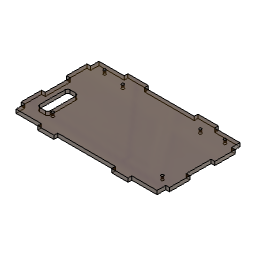
PCB Plate (Autodesk Fusion 360 design; units mm, degrees)
Autodesk Fusion 360 part; units mm, degrees
sketch "Sketch1" plane through (0, 0, 0) normal (0, 0, 1) x (1, 0, 0)
  line L0 (90, -52.5) -> (-90, -52.5)
  line L1 (-90, -52.5) -> (-90, 52.5)
  line L2 (-90, 52.5) -> (90, 52.5)
  line L3 (90, 52.5) -> (90, -52.5)
  line L4 (90, -52.5) -> (-90, 52.5) construction
  line L5 (-90, -52.5) -> (90, 52.5) construction
  line L6 (-85.5, 52.5) -> (-85.5, -52.5)
  line L7 (85.5, 52.5) -> (85.5, -52.5)
  line L8 (-90, -48) -> (90, -48)
  line L9 (-90, -52.5) -> (-55, -52.5)
  line L10 (-55, -52.5) -> (-55, -48)
  line L11 (-55, -48) -> (-90, -48)
  line L12 (-90, -48) -> (-90, -52.5)
  line L13 (-55, -52.5) -> (-35, -52.5)
  line L14 (-35, -52.5) -> (-35, -48)
  line L15 (-35, -48) -> (-55, -48)
  line L16 (-55, -48) -> (-55, -52.5)
  line L17 (90, -52.5) -> (55, -52.5)
  line L18 (55, -52.5) -> (55, -48)
  line L19 (55, -48) -> (90, -48)
  line L20 (90, -48) -> (90, -52.5)
  line L21 (-90, -52.5) -> (-85.5, -52.5)
  line L22 (-85.5, -52.5) -> (-85.5, -37.5)
  line L23 (-85.5, -37.5) -> (-90, -37.5)
  line L24 (-90, -37.5) -> (-90, -52.5)
  line L25 (90, -52.5) -> (85.5, -52.5)
  line L26 (85.5, -52.5) -> (85.5, -37.5)
  line L27 (85.5, -37.5) -> (90, -37.5)
  line L28 (90, -37.5) -> (90, -52.5)
  line L29 (-85.5, -37.5) -> (-90, -37.5)
  line L30 (-90, -37.5) -> (-90, -12.5)
  line L31 (-90, -12.5) -> (-85.5, -12.5)
  line L32 (-85.5, -12.5) -> (-85.5, -37.5)
  line L33 (90, -37.5) -> (85.5, -37.5)
  line L34 (85.5, -37.5) -> (85.5, -12.5)
  line L35 (85.5, -12.5) -> (90, -12.5)
  line L36 (90, -12.5) -> (90, -37.5)
  line L37 (-85.5, -12.5) -> (-90, -12.5)
  line L38 (-90, -12.5) -> (-90, 17.5)
  line L39 (-90, 17.5) -> (-85.5, 17.5)
  line L40 (-85.5, 17.5) -> (-85.5, -12.5)
  line L41 (-85.5, 17.5) -> (-90, 17.5)
  line L42 (-90, 17.5) -> (-90, 42.5)
  line L43 (-90, 42.5) -> (-85.5, 42.5)
  line L44 (-85.5, 42.5) -> (-85.5, 17.5)
  line L45 (90, -12.5) -> (85.5, -12.5)
  line L46 (85.5, -12.5) -> (85.5, 17.5)
  line L47 (85.5, 17.5) -> (90, 17.5)
  line L48 (90, 17.5) -> (90, -12.5)
  line L49 (90, 17.5) -> (85.5, 17.5)
  line L50 (85.5, 17.5) -> (85.5, 42.5)
  line L51 (85.5, 42.5) -> (90, 42.5)
  line L52 (90, 42.5) -> (90, 17.5)
  line L53 (55, -52.5) -> (35, -52.5)
  line L54 (35, -52.5) -> (35, -48)
  line L55 (35, -48) -> (55, -48)
  line L56 (55, -48) -> (55, -52.5)
  line L57 (-90, 43) -> (90, 43) construction
  line L58 (0, 43) -> (0, 40) construction
  circle A0 centre (47, 43) radius 1.6
  circle A1 centre (-47, 43) radius 1.6
  line L59 (-90, 47) -> (90, 47) construction
  circle A2 centre (73, 47) radius 1.6
  circle A3 centre (-73, 47) radius 1.6
  circle A4 centre (73, -29) radius 1.6
  circle A5 centre (-60, -29) radius 1.6
  line L60 (-66, -32) -> (-73, -32)
  line L61 (-76, -29) -> (-76, 2)
  line L62 (-73, 5) -> (-66, 5)
  line L63 (-63, 2) -> (-63, -29)
  line L64 (-63, -32) -> (-76, 5) construction
  line L65 (-76, -32) -> (-63, 5) construction
  arc A6 (-63, 2) -> (-66, 5) centre (-66, 2) ccw
  arc A7 (-73, 5) -> (-76, 2) centre (-73, 2) ccw
  arc A8 (-76, -29) -> (-73, -32) centre (-73, -29) ccw
  arc A9 (-66, -32) -> (-63, -29) centre (-66, -29) ccw
  line L66 (-55, 52.5) -> (-30, 52.5)
  line L67 (-30, 52.5) -> (-30, 57)
  line L68 (-30, 57) -> (-55, 57)
  line L69 (-55, 57) -> (-55, 52.5)
  line L70 (30, 52.5) -> (55, 52.5)
  line L71 (55, 52.5) -> (55, 57)
  line L72 (55, 57) -> (30, 57)
  line L73 (30, 57) -> (30, 52.5)
  point P0 (-69.5, -13.5)
  dimension "d1" = 180
  dimension "d2" = 105
  dimension "d3" = 4.5
  dimension "d4" = 4.5
  dimension "d5" = 4.5
  dimension "d6" = 35
  dimension "d7" = 20
  dimension "d8" = 35
  dimension "d10" = 15
  dimension "d11" = 15
  dimension "d12" = 25
  dimension "d13" = 25
  dimension "d14" = 30
  dimension "d15" = 25
  dimension "d16" = 30
  dimension "d17" = 25
  dimension "d18" = 20
  dimension "d20" = 91
  dimension "d21" = 3.2
  dimension "d22" = 3.2
  dimension "d23" = 47
  dimension "d24" = 47
  dimension "d25" = 4
  dimension "d26" = 3.2
  dimension "d27" = 3.2
  dimension "d28" = 73
  dimension "d29" = 73
  dimension "d30" = 3.2
  dimension "d31" = 72
  dimension "d32" = 3.2
  dimension "d33" = 72
  dimension "d34" = 60
  dimension "d35" = 13
  dimension "d36" = 37
  dimension "d37" = 3
  dimension "d38" = 3
  dimension "d39" = 3
  dimension "d40" = 3
  dimension "d41" = 3
  dimension "d42" = 3
  dimension "d48" = 25
  dimension "d49" = 4.5
  dimension "d50" = 25
  dimension "d51" = 4.5
  dimension "d52" = 35
  dimension "d53" = 35
  constraint horizontal L0
  constraint perpendicular L0 L1
  constraint parallel L0 L2
  constraint parallel L1 L3
  constraint coincident L4 origin
  constraint coincident L5 origin
  constraint coincident L2 L6.start
  constraint coincident L0 L6.end
  constraint perpendicular L0 L6
  constraint coincident L2 L7.start
  constraint coincident L0 L7.end
  constraint perpendicular L0 L7
  constraint coincident L1 L8.start
  constraint coincident L3 L8.end
  constraint perpendicular L3 L8
  constraint horizontal L9
  constraint vertical L10
  constraint horizontal L11
  constraint vertical L12
  constraint horizontal L13
  constraint vertical L14
  constraint horizontal L15
  constraint vertical L16
  constraint horizontal L17
  constraint vertical L18
  constraint horizontal L19
  constraint vertical L20
  constraint horizontal L21
  constraint vertical L22
  constraint horizontal L23
  constraint vertical L24
  constraint horizontal L25
  constraint vertical L26
  constraint horizontal L27
  constraint vertical L28
  constraint horizontal L29
  constraint vertical L30
  constraint horizontal L31
  constraint vertical L32
  constraint horizontal L33
  constraint vertical L34
  constraint horizontal L35
  constraint vertical L36
  constraint horizontal L37
  constraint vertical L38
  constraint horizontal L39
  constraint vertical L40
  constraint horizontal L41
  constraint vertical L42
  constraint horizontal L43
  constraint vertical L44
  constraint horizontal L45
  constraint vertical L46
  constraint horizontal L47
  constraint vertical L48
  constraint horizontal L49
  constraint vertical L50
  constraint horizontal L51
  constraint vertical L52
  constraint horizontal L53
  constraint vertical L54
  constraint horizontal L55
  constraint vertical L56
  constraint coincident L1 L57.start
  constraint coincident L42 L57.start
  constraint coincident L52 L57.end
  constraint perpendicular L52 L57
  constraint midpoint L57 L58.start
  constraint perpendicular L57 L58
  constraint coincident L57 A0.centre
  constraint coincident L57 A1.centre
  constraint coincident L1 L59.start
  constraint coincident L3 L59.end
  constraint perpendicular L3 L59
  constraint coincident L59 A2.centre
  constraint coincident L59 A3.centre
  constraint vertical A2.centre A4.centre
  constraint horizontal L60
  constraint perpendicular L60 L61
  constraint parallel L60 L62
  constraint parallel L61 L63
  constraint coincident L64 P0
  constraint coincident L65 P0
  constraint coincident L65.end L62
  constraint coincident L65.end L63
  constraint tangent L62 A6
  constraint tangent L63 A6
  constraint coincident L64.end L62
  constraint coincident L64.end L61
  constraint tangent L62 A7
  constraint tangent L61 A7
  constraint coincident L65.start L61
  constraint coincident L65.start L60
  constraint tangent L61 A8
  constraint tangent L60 A8
  constraint coincident L64.start L63
  constraint coincident L64.start L60
  constraint tangent L63 A9
  constraint tangent L60 A9
  constraint horizontal L66
  constraint vertical L67
  constraint horizontal L68
  constraint vertical L69
  constraint coincident L2 L66.start
  constraint horizontal L70
  constraint vertical L71
  constraint horizontal L72
  constraint vertical L73
  constraint coincident L2 L70.start
  measures "d1" distance of L1.end L2.end
  measures "d2" distance of L0.end L1.end
  measures "d3" distance of L3 L7
  measures "d4" distance of L1 L6
  measures "d5" distance of L0 L8
  measures "d6" distance of L0.end L9.end
  measures "d7" distance of L9.end L13.end
  measures "d8" distance of L0.start L17.end
  measures "d10" distance of L0.end L23.end
  measures "d11" distance of L0.start L27.end
  measures "d12" distance of L22.end L31.end
  measures "d13" distance of L27.end L35.end
  measures "d14" distance of L31.end L39.end
  measures "d15" distance of L39.end L43.end
  measures "d16" distance of L35.end L47.end
  measures "d17" distance of L47.end L51.end
  measures "d18" distance of L17.end L53.end
  measures "d20" distance of L8 L57
  measures "d21" diameter of A0
  measures "d22" diameter of A1
  measures "d23" horizontal distance of L58.end A0.centre
  measures "d24" distance of L58 A1.centre
  measures "d25" distance of L57 L59
  measures "d26" diameter of A2
  measures "d27" diameter of A3
  measures "d28" distance of L58 A2.centre
  measures "d29" distance of L58 A3.centre
  measures "d30" diameter of A4
  measures "d31" distance of L57 A4.centre
  measures "d32" diameter of A5
  measures "d33" distance of L57 A5.centre
  measures "d34" distance of L58 A5.centre
  measures "d35" distance of L64.end L65.end
  measures "d36" distance of L65.start L64.end
  measures "d37" distance of A5.centre L63
  measures "d38" distance of A5.centre L60
  measures "d39" radius of A6
  measures "d40" radius of A7
  measures "d41" radius of A8
  measures "d42" radius of A9
  measures "d48" distance of L66.start L66.end
  measures "d49" distance of L66.start L68.end
  measures "d50" distance of L70.start L70.end
  measures "d51" distance of L70.start L72.end
  measures "d52" distance of L3 L71
  measures "d53" distance of L1 L69
extrude "Extrude1" add sketch "Sketch1" along normal blind 4.5 contours L0 L8 L18 L53 L54 L55 L56 | L2 L6 L7 L8 L11 L15 L19 L22 L26 L32 L34 L40 L44 L46 L50 L55 L66 L70 | L3 L7 L27 L33 L34 L35 L36 L45 | L0 L8 L10 L13 L14 L15 L16 | L3 L7 L47 L49 L50 L51 L52 | L1 L6 L23 L29 L30 L31 L32 L37 | L2 L70 L71 L72 L73 | L1 L6 L39 L41 L42 L43 L44 | L2 L66 L67 L68 L69
move_face "OffsetFaces1" offset -0.1 4 faces at (55, -51, 1.5) (-35, -51, 1.5) (-30, 54, 1.5) (55, 54, 1.5)
move_face "OffsetFaces2" offset -0.1 4 faces at (35, -51, 1.5) (-55, -51, 1.5) (30, 55.5, 1.5) (-55, 55.5, 1.5)
move_face "OffsetFaces3" offset -0.1 4 faces at (-88.5, 17.5, 1.5) (-87, -37.5, 1.5) (87, -37.5, 1.5) (87, 17.5, 1.5)
move_face "OffsetFaces4" offset -0.1 4 faces at (-88.5, 42.5, 1.5) (-88.5, -12.5, 1.5) (87, 42.5, 1.5) (87, -12.5, 1.5)
equation "TabRelief = -0.1 mm"
equation "d55 = TabRelief"
equation "d56 = TabRelief"
equation "d57 = TabRelief"
equation "d58 = TabRelief"
